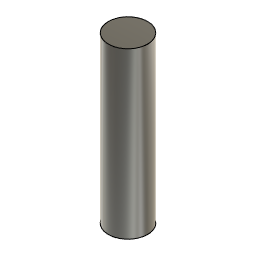
CILINDRO DE UNION v3 (Autodesk Fusion 360 design; units mm, degrees)
Autodesk Fusion 360 part; units mm, degrees
cylinder "CilindroPrimitivo1" add diameter 10 height 42 placed x (1, 0, 0) y (0, 1, 0) z (0, 0, 1) at (0, 0, 0)
